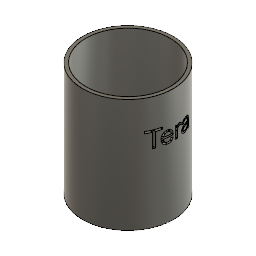
笔筒 (Autodesk Fusion 360 design; units mm, degrees)
Autodesk Fusion 360 part; units mm, degrees
note: some values were not read from the file. Chosen so that the rebuilt part matches the saved one: which bodies a step acts on; which face or edge a step refers to; the layout of a text.
cylinder "圆柱体基本要素1" add diameter 80 height 100 placed x (1, 0, 0) y (0, 0, -1) z (0, 1, 0) at (0, 0, 0) makes body 1
shell "抽壳1" thickness 3 removed faces 1 at (9.4847, 100, 14.2223) on bodies 1
sketch "草图2" plane through (0, 0, 0) normal (1, 0, 0) x (0, 0, -1)
  line L0 (90, 60) -> (127.5879, 60) construction
  line L1 (127.5879, 60) -> (127.5879, 80) construction
  line L2 (127.5879, 80) -> (90, 80) construction
  line L3 (90, 80) -> (90, 60) construction
  text T0 "Tera" font "Arial" height 20 align ink ink in box 0 x 0 at (90.01, 60.02) x (1, 0) y (0, 1) spacing 1 kerned height is em
extrude "拉伸1" add sketch "草图2" along normal blind 60 separate body text T0 makes body 2 at (20, 63.7114, -111.9631) makes body 3 at (20, 64.9907, -107.2463) makes body 4 at (30, 66.3079, -122.7484) makes body 5 at (40, 64.4634, -94.7268)
move_body "移动1" bodies 2 5 4 3 to x (1, 0, 0) y (0, 1, 0) z (0, 0, 1) at (0, 0, 110)
combine "合并1" operation cut target body 1 tool bodies 5 3 4 2 makes body 6 at (35.0483, 63.3225, -11.8581) makes body 7 at (37.3076, 66.436, 7.1737)
